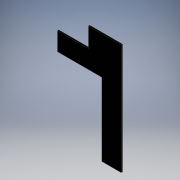
# Autodesk Inventor part: BA03
Saved by Autodesk Inventor 2017 (Build 210142000, 142)
## iProperties
Created: 2018-10-18
Part Number: BA03
Material: ABS Plastic
Document SubType Name: Modeling
Designer: Dell
Density: 1.06 g/cm^3
Appearance: Smooth - Black
Author: Dell
Autodesk Inventor part; units mm, degrees
ref_plane "YZ Plane" through (0, 0, 0) normal (1, 0, 0) x (0, 1, 0)
ref_plane "XZ Plane" through (0, 0, 0) normal (0, 1, 0) x (-1, 0, 0)
ref_plane "XY Plane" through (0, 0, 0) normal (0, 0, 1) x (1, 0, 0)
sketch "Sketch1" plane through (0, 0, 0) normal (0, 0, 1) x (1, 0, 0)
  line L0 (0, 0) -> (307.2255, 0)
  line L1 (307.2255, 0) -> (307.2255, -177.8)
  line L2 (307.2255, -177.8) -> (0, -177.8)
  line L3 (0, -177.8) -> (0, 0)
  line L4 (460.8382, 266.0651) -> (307.2255, 0)
  line L5 (307.2255, 0) -> (0, 0)
  line L6 (0, 0) -> (-153.6127, 266.0651)
  line L7 (-153.6127, 266.0651) -> (0, 532.1302)
  line L8 (0, 532.1302) -> (307.2255, 532.1302)
  line L9 (307.2255, 532.1302) -> (460.8382, 266.0651)
  point P0 (153.6127, 266.0651)
  dimension "d1" = 177.8
  dimension "d37" = 307.2255
  constraints: 20 end point, 2 parallel, 1 horizontal, 1 perpendicular, 13 other
  measures "d1" distance of L0.end L1.end
  measures "d37" distance of L0.start L0.end
extrude "Extrusion1" add sketch "Sketch1" along normal blind 6.35 contours L0 L1 L2 L3
sketch "Sketch2" plane through (0, 0, 0) normal (0, 1, 0) x (1, 0, 0)
  line L0 (307.2255, -6.35) -> (0, -6.35) projected
  line L1 (0, -6.35) -> (-3.6662, -6.35)
  line L2 (-3.6662, -6.35) -> (0, 0)
  line L3 (0, 0) -> (0, -6.35) projected
  line L4 (0, 0) -> (0, -6.35) projected
  line L5 (0, -6.35) -> (0, 0)
  line L6 (307.2255, -6.35) -> (310.8917, -6.35)
  line L7 (307.2255, 0) -> (307.2255, -6.35) projected
  line L8 (310.8917, -6.35) -> (307.2255, 0)
  line L9 (307.2255, 0) -> (307.2255, -6.35)
  dimension "d4" = 30
  dimension "d5" = 60
  constraints: 12 end point, 2 collinear, 2 horizontal
  measures "d4" angle of L3 L2
  measures "d5" angle of L6 L8
extrude "Extrusion2" add sketch "Sketch2" against normal blind 177.8
sketch "Sketch3" plane through (0, 0, 6.35) normal (0, 0, 1) x (1, 0, 0)
  line L0 (25.8917, -88.9) -> (225.8917, -88.9)
  line L1 (225.8917, -88.9) -> (225.8917, 0)
  line L2 (225.8917, 0) -> (25.8917, 0)
  line L3 (25.8917, 0) -> (25.8917, -88.9)
  line L4 (-3.6662, 0) -> (310.8917, 0) projected
  line L5 (25.8917, -88.9) -> (150.8917, -88.9)
  line L6 (150.8917, -88.9) -> (150.8917, 0)
  line L7 (150.8917, 0) -> (25.8917, 0)
  line L8 (25.8917, 0) -> (25.8917, -88.9)
  line L9 (310.8917, 0) -> (310.8917, -177.8) projected
  point P0 (0, 0)
  point P1 (153.6127, 0)
  dimension "d8" = 200
  dimension "d9" = 88.9
  dimension "d30" = 75
  dimension "d31" = 85
  constraints: 16 end point, 4 parallel, 2 horizontal, 2 perpendicular, 2 point on line, 1 midpoint
  measures "d8" distance of L1.end L2.end
  measures "d9" distance of L0.end L1.end
  measures "d30" distance between parallel lines of L1 L6
  measures "d31" distance between parallel lines of L9 L1
extrude "Extrusion3" cut sketch "Sketch3" against normal through all contours L3 L2 L6 L0
sketch "Sketch5" plane through (0, 0, 6.35) normal (0, 0, 1) x (1, 0, 0)
  line L0 (310.8917, 0) -> (310.8917, -177.8) projected
  line L1 (310.8917, -177.8) -> (215.6417, -177.8)
  line L2 (215.6417, -177.8) -> (215.6417, -533.4)
  line L3 (215.6417, -533.4) -> (310.8917, -533.4)
  line L4 (310.8917, -533.4) -> (310.8917, -177.8)
  point P0 (0, 0)
  dimension "d20" = 95.25
  dimension "d21" = 355.6
  constraints: 8 end point, 2 parallel, 1 horizontal, 1 perpendicular
  measures "d20" distance of L3.end L2.end
  measures "d21" distance of L2.end L1.end
extrude "Extrusion5" add sketch "Sketch5" against normal blind 10
sketch "Sketch7" plane through (307.2255, -177.8, 0) normal (0, 1, 0) x (1, 0, 0)
  line L0 (0, 0) -> (3.6662, -6.35) projected
  line L1 (3.6662, -6.35) -> (3.6662, 3.65) projected
  line L2 (-91.5838, 3.65) -> (3.6662, 3.65) projected
  line L3 (-91.5838, 0) -> (-91.5838, 3.65) projected
  line L4 (0, 0) -> (-91.5838, 0) projected
  point P0 (-307.2255, 0)
extrude "Extrusion6" cut sketch "Sketch7" against normal through all
sketch "Sketch9" plane through (0, 0, 6.35) normal (0, 0, 1) x (1, 0, 0)
  line L0 (-3.6662, 0) -> (25.8917, 0) projected
  line L1 (25.8917, -88.9) -> (-3.6662, -88.9)
  line L2 (-3.6662, -88.9) -> (-3.6662, 0)
  line L3 (-3.6662, 0) -> (25.8917, 0)
  line L4 (25.8917, 0) -> (25.8917, -88.9)
  point P0 (0, 0)
  constraints: 8 end point, 2 parallel, 1 horizontal, 1 perpendicular
extrude "Extrusion8" cut sketch "Sketch9" against normal through all
sketch "Sketch10" plane through (150.8917, 0, 0) normal (0, 1, 0) x (1, 0, 0)
  line L0 (0, -6.35) -> (-154.5578, -6.35) projected
  line L1 (-150.8917, 0) -> (-154.5578, 0)
  line L2 (-154.5578, 0) -> (-154.5578, -6.35)
  line L3 (-154.5578, -6.35) -> (-150.8917, -6.35)
  line L4 (-150.8917, -6.35) -> (-150.8917, 0)
  line L5 (160, -6.35) -> (156.3338, 0) projected
  line L6 (156.3338, 0) -> (160, 0)
  line L7 (160, 0) -> (160, -6.35)
  line L8 (160, -6.35) -> (156.3338, -6.35)
  line L9 (156.3338, -6.35) -> (156.3338, 0)
  constraints: 16 end point, 4 parallel, 2 horizontal, 2 perpendicular
extrude "Extrusion9" cut sketch "Sketch10" against normal through all
sketch "Sketch11" plane through (0, 0, 6.35) normal (0, 0, 1) x (1, 0, 0)
  line L0 (150.8917, 0) -> (307.2255, 0) projected
  line L1 (307.2255, 0) -> (310.8917, 0)
  line L2 (310.8917, 0) -> (310.8917, -533.4)
  line L3 (310.8917, -533.4) -> (307.2255, -533.4)
  line L4 (307.2255, -533.4) -> (307.2255, 0)
  line L5 (215.6417, -177.8) -> (215.6417, -533.4) projected
  point P0 (0, 0)
  dimension "d38" = 95.25
  constraints: 8 end point, 2 parallel, 1 coincident, 1 horizontal, 1 perpendicular
  measures "d38" distance between parallel lines of L5 L2
extrude "Extrusion10" add sketch "Sketch11" against normal blind 6.35
sketch "Sketch12" plane through (0, 0, 6.35) normal (0, 0, 1) x (1, 0, 0)
  line L0 (150.8917, 0) -> (310.8917, 0) projected
  line L1 (150.8917, 0) -> (310.8917, 0)
  line L2 (310.8917, 0) -> (310.8917, 6.35)
  line L3 (310.8917, 6.35) -> (150.8917, 6.35)
  line L4 (150.8917, 6.35) -> (150.8917, 0)
  point P0 (0, 0)
  point P1 (310.8917, 3.175)
  dimension "d41" = 6.35
  constraints: 8 end point, 2 parallel, 1 horizontal, 1 midpoint, 1 perpendicular, 1 vertical alignment
  measures "d41" distance of L3.end L0.start
extrude "Extrusion11" add sketch "Sketch12" against normal blind 6.35
body "Solid1"
